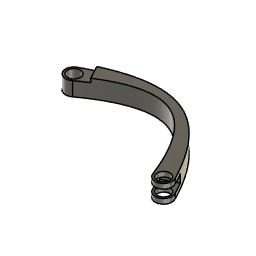
proximal_finger (Autodesk Fusion 360 archive; units mm, degrees)
design "fixador_final_pa"
Autodesk Fusion 360 part; units mm, degrees
sketch "Esboço1" plane through (0, 0, 0) normal (0, 0, 1) x (1, 0, 0)
  circle A0 centre (42.203, 3.5284) radius 3.25
  circle A1 centre (-10.898, 22.0884) radius 3.25
  spline S0 degree 5 poles (-12.8734, 24.6692) (-11.3777, 25.4931) (-8.4159, 27.0342) (-4.0626, 29.0252) (1.5602, 31.0283) (8.2656, 32.3731) (14.6199, 32.4582) (20.5957, 31.1854) (26.1805, 28.5094) (31.3923, 24.4956) (36.2604, 19.2489) (39.9032, 14.1482) (42.5027, 9.8471) (44.1777, 6.7718) (45.0008, 5.1822) knots 0 0 0 0 0 0 0.1 0.2 0.3 0.4 0.5 0.6 0.7 0.8 0.9 1 1 1 1 1 1
  spline S1 degree 5 poles (-8.8814, 19.5398) (-7.5737, 20.4865) (-4.9887, 22.2654) (-1.203, 24.5904) (3.6582, 26.9923) (9.4033, 28.7533) (14.7887, 29.1675) (19.7872, 28.1329) (24.3882, 25.6093) (28.6117, 21.6721) (32.4881, 16.4352) (35.3354, 11.2947) (37.3372, 6.939) (38.6133, 3.8164) (39.2367, 2.2004) knots 0 0 0 0 0 0 0.1 0.2 0.3 0.4 0.5 0.6 0.7 0.8 0.9 1 1 1 1 1 1
  point P0 (20, 31)
  point P1 (19, 28)
  dimension "d1" = 6.5
  dimension "d4" = 6.5
  dimension "d5" = 18.56
  constraint coincident A1 S0.start
  constraint coincident A1 S1.start
  constraint coincident S0.end A0
  constraint coincident S1.end A0
  measures "d1" diameter of A0
  measures "d4" diameter of A1
  measures "d5" vertical distance of A0.centre A1.centre
extrude "Extrusão1" add sketch "Esboço1" along normal blind 6.9 contours A0 S1 | A0 A1 S0 S1 | A1 S0 picked at (41.2142, 3.6571) picked at (-12.2396, 22.8854)
ref_plane "Plano de trabalho1" through (45.0008, 5.1822, 6.9) normal (0.888029, 0.459787, 0) x (-0.459787, 0.888029, 0)
sketch "Esboço2" plane through (37.6033, 19.4696, 0) normal (0.888029, 0.459787, 0) x (-0.459787, 0.888029, 0)
  line L0 (-11.004, 1.9057, -0.1252) -> (-21.2031, 1.9057, -0.1252)
  line L1 (-21.2031, 1.9057, -0.1252) -> (-21.2031, 5.0057, -0.1252)
  line L2 (-21.2031, 5.0057, -0.1252) -> (-11.004, 5.0057, -0.1252)
  line L3 (-11.004, 5.0057, -0.1252) -> (-11.004, 1.9057, -0.1252)
  line L4 (-14.6648, 0.0065, -0.0718) -> (-14.6648, 7.5657, -0.0718)
  dimension "d8" = 3.1
  dimension "d16" = 1.9
extrude "Extrusão2" cut sketch "Esboço2" against normal blind 8 contours L0 L1 L2 L3 in plane through (37.4922, 19.412, 0) normal (0.888029, 0.459787, 0)
extrude "Extrusão3" cut sketch "Esboço2" along normal blind 4 contours L0 L1 L2 L3 in plane through (37.4922, 19.412, 0) normal (0.888029, 0.459787, 0)
hole "Furo1" at (42.203, 3.5284, 6.9) direction (0, 0, -1) diameter 5 depth 10 tip angle 118
ref_plane "Plano de trabalho2" through (-11.9899, 25.1496, 0) normal (-0.47273, 0.881208, 0) x (-0.881208, -0.47273, 0)
sketch "Esboço3" plane through (-13.156, 24.5239, 0) normal (-0.47273, 0.881208, 0) x (-0.881208, -0.47273, 0)
  line L0 (-6.4299, 5.4, -0.1555) -> (3.9958, 5.4, -0.1555)
  line L1 (3.9958, 5.4, -0.1555) -> (3.9958, 6.9, -0.1555)
  line L2 (3.9958, 6.9, -0.1555) -> (-6.4299, 6.9, -0.1555)
  line L3 (-6.4299, 6.9, -0.1555) -> (-6.4299, 5.4, -0.1555)
  dimension "d17" = 1.5
  dimension "d18" = 5.4
extrude "Extrusão4" cut sketch "Esboço3" against normal blind 9 contours L0 L1 L2 L3 in plane through (-13.0825, 24.3869, 0) normal (-0.47273, 0.881208, 0)
extrude "Extrusão5" cut sketch "Esboço3" along normal blind 3 contours L0 L1 L2 L3 in plane through (-13.0825, 24.3869, 0) normal (-0.47273, 0.881208, 0)
hole "Furo2" at (-10.898, 22.0884, 0) direction (0, 0, 1) diameter 5 depth 10 tip angle 118

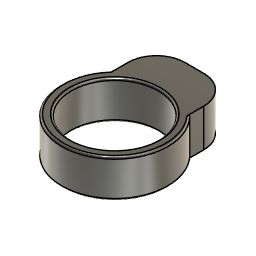
design "anel_final"
Autodesk Fusion 360 part; units mm, degrees
sketch "Esboço1" plane through (0, 0, 0) normal (0, 0, 1) x (1, 0, 0)
  circle A0 centre (0, 0) radius 11.5
  circle A1 centre (0, 0) radius 14
  line L0 (-10, 9.798) -> (-10, 21)
  line L1 (-10, 21) -> (10, 21)
  line L2 (10, 21) -> (10, 9.798)
  line L3 (0, 0) -> (0, 14)
  dimension "d1" = 23
  dimension "d2" = 28
  dimension "d3" = 20
  dimension "d5" = 7
  constraint coincident A0.centre A1.centre
  constraint coincident A1 L0.start
  constraint vertical L0
  constraint perpendicular L0 L1
  constraint coincident A1 L2.end
  constraint perpendicular L1 L2
  constraint coincident A1 L3.end
  constraint vertical L3
  measures "d1" diameter of A0
  measures "d2" diameter of A1
  measures "d3" distance of L0 L2
  measures "d5" distance of L1 L3.end
extrude "Extrusão1" add sketch "Esboço1" along normal blind 10
hole "Furo1" at (0, 21, 5) direction (0, -1, 0) diameter 2.8 depth 5.5 tip angle 180
fillet "Arredondamento1" radius 0.5 4 edges at (-10.7218, 4.1586, 10) (-10.7218, 4.1586, 0) (0, -14, 0) (0, -14, 10)
fillet "Arredondamento2" radius 7.5 2 edges at (-10, 21, 5) (10, 21, 5)
